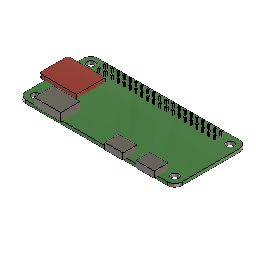
PiZero (Autodesk Fusion 360 design; units mm, degrees)
Autodesk Fusion 360 part; units mm, degrees
sketch "Skizze1" plane through (0, 0, 0) normal (0, 0, 1) x (1, 0, 0)
  line L0 (0, 0) -> (65, 0)
  line L1 (65, 0) -> (65, 30)
  line L2 (65, 30) -> (0, 30)
  line L3 (0, 30) -> (0, 0)
  dimension "d1" = 65
  dimension "d2" = 30
  constraint horizontal L0
  constraint vertical L1
  constraint horizontal L2
  constraint vertical L3
  constraint coincident L0.start L3.end
  measures "d1" distance of L0.start L0.end
  measures "d2" distance of L0.end L1.end
extrude "Extrusion1" add sketch "Skizze1" along normal blind 1.3
fillet "Abrundung1" radius 3 4 edges at (65, 0, 0.65) (0, 0, 0.65) (0, 30, 0.65) (65, 30, 0.65)
sketch "Skizze2" plane through (0, 0, 1.3) normal (0, 0, 1) x (-1, 0, 0)
  arc A0 (-65, -27) -> (-62, -30) centre (-62, -27) ccw
  line L0 (-62, -30) -> (-3, -30)
  arc A1 (-3, -30) -> (0, -27) centre (-3, -27) ccw
  line L1 (0, -27) -> (0, -3)
  arc A2 (0, -3) -> (-3, 0) centre (-3, -3) ccw
  line L2 (-3, 0) -> (-62, 0)
  arc A3 (-62, 0) -> (-65, -3) centre (-62, -3) ccw
  line L3 (-65, -3) -> (-65, -27)
  line L4 (2.5, -23) -> (-13, -23)
  line L5 (-13, -23) -> (-13, -11)
  line L6 (-13, -11) -> (2.5, -11)
  line L7 (2.5, -11) -> (2.5, -23)
  dimension "d7" = 12
  dimension "d8" = 15.5
  dimension "d9" = 7
  dimension "d10" = 2.5
  constraint horizontal L4
  constraint vertical L5
  constraint horizontal L6
  constraint vertical L7
  measures "d7" distance of L4.end L5.end
  measures "d8" distance of L5.end L6.end
  measures "d9" distance of L0 L4
  measures "d10" distance of L1 L7
extrude "Extrusion2" add sketch "Skizze2" along normal blind 1.5 contours L1 L4 L5 L6 | L1 L4 L6 L7
fillet "Abrundung2" radius 1 2 edges at (-2.5, 11, 2.05) (-2.5, 23, 2.05)
sketch "Skizze3" plane through (0, 0, 1.3) normal (0, 0, 1) x (-1, 0, 0)
  line L0 (-13, -11) -> (0, -11)
  line L1 (0, -11) -> (0, -3)
  arc A0 (0, -3) -> (-3, 0) centre (-3, -3) ccw
  line L2 (-3, 0) -> (-62, 0)
  arc A1 (-62, 0) -> (-65, -3) centre (-62, -3) ccw
  line L3 (-65, -3) -> (-65, -27)
  arc A2 (-65, -27) -> (-62, -30) centre (-62, -27) ccw
  line L4 (-62, -30) -> (-3, -30)
  arc A3 (-3, -30) -> (0, -27) centre (-3, -27) ccw
  line L5 (0, -27) -> (0, -23)
  line L6 (0, -23) -> (-13, -23)
  line L7 (-13, -23) -> (-13, -11)
  line L8 (-7, -7.5) -> (-18, -7.5)
  line L9 (-18, -7.5) -> (-18, 0.5)
  line L10 (-18, 0.5) -> (-7, 0.5)
  line L11 (-7, 0.5) -> (-7, -7.5)
  dimension "d15" = 8
  dimension "d16" = 11
  dimension "d17" = 7
  dimension "d18" = 0.5
  constraint horizontal L8
  constraint vertical L9
  constraint horizontal L10
  constraint vertical L11
  measures "d15" distance of L8.end L9.end
  measures "d16" distance of L9.end L10.end
  measures "d17" distance of L1 L11
  measures "d18" distance of L2 L10
extrude "Extrusion3" add sketch "Skizze3" along normal blind 3.2 contours L2 L8 L9 L11 | L2 L9 L10 L11
sketch "Skizze4" plane through (0, 0, 1.3) normal (0, 0, 1) x (-1, 0, 0)
  line L0 (-18, -7.5) -> (-18, 0)
  line L1 (-18, 0) -> (-62, 0)
  arc A0 (-62, 0) -> (-65, -3) centre (-62, -3) ccw
  line L2 (-65, -3) -> (-65, -27)
  arc A1 (-65, -27) -> (-62, -30) centre (-62, -27) ccw
  line L3 (-62, -30) -> (-3, -30)
  arc A2 (-3, -30) -> (0, -27) centre (-3, -27) ccw
  line L4 (0, -27) -> (0, -23)
  line L5 (0, -23) -> (-13, -23)
  line L6 (-13, -23) -> (-13, -11)
  line L7 (-13, -11) -> (0, -11)
  line L8 (0, -11) -> (0, -3)
  arc A3 (0, -3) -> (-3, 0) centre (-3, -3) ccw
  line L9 (-3, 0) -> (-7, 0)
  line L10 (-7, 0) -> (-7, -7.5)
  line L11 (-7, -7.5) -> (-18, -7.5)
  line L12 (-37.4, -4.2) -> (-44.9, -4.2)
  line L13 (-44.9, -4.2) -> (-44.9, 1.5)
  line L14 (-44.9, 1.5) -> (-37.4, 1.5)
  line L15 (-37.4, 1.5) -> (-37.4, -4.2)
  dimension "d21" = 7.5
  dimension "d22" = 5.7
  dimension "d23" = 37.4
  dimension "d24" = 1.5
  constraint horizontal L12
  constraint vertical L13
  constraint horizontal L14
  constraint vertical L15
  measures "d21" distance of L13.end L14.end
  measures "d22" distance of L12.end L13.end
  measures "d23" distance of L8 L15
  measures "d24" distance of L1 L14
extrude "Extrusion4" add sketch "Skizze4" along normal blind 2.6 contours L1 L12 L13 L15 | L1 L13 L14 L15
pattern_linear "R-Anordnung1" count 2 spacing 13 along (1, 0, 0) of "Extrusion4"
sketch "Skizze5" plane through (0, 0, 1.3) normal (0, 0, 1) x (-1, 0, 0)
  line L0 (-50.4, 0) -> (-50.4, -4.2)
  line L1 (-50.4, -4.2) -> (-57.9, -4.2)
  line L2 (-57.9, -4.2) -> (-57.9, 0)
  line L3 (-57.9, 0) -> (-62, 0)
  arc A0 (-62, 0) -> (-65, -3) centre (-62, -3) ccw
  line L4 (-65, -3) -> (-65, -27)
  arc A1 (-65, -27) -> (-62, -30) centre (-62, -27) ccw
  line L5 (-62, -30) -> (-3, -30)
  arc A2 (-3, -30) -> (0, -27) centre (-3, -27) ccw
  line L6 (0, -27) -> (0, -23)
  line L7 (0, -23) -> (-13, -23)
  line L8 (-13, -23) -> (-13, -11)
  line L9 (-13, -11) -> (0, -11)
  line L10 (0, -11) -> (0, -3)
  arc A3 (0, -3) -> (-3, 0) centre (-3, -3) ccw
  line L11 (-3, 0) -> (-7, 0)
  line L12 (-7, 0) -> (-7, -7.5)
  line L13 (-7, -7.5) -> (-18, -7.5)
  line L14 (-18, -7.5) -> (-18, 0)
  line L15 (-18, 0) -> (-37.4, 0)
  line L16 (-37.4, 0) -> (-37.4, -4.2)
  line L17 (-37.4, -4.2) -> (-44.9, -4.2)
  line L18 (-44.9, -4.2) -> (-44.9, 0)
  line L19 (-44.9, 0) -> (-50.4, 0)
  point P0 (-3.5, -26.5)
  point P1 (-61.5, -26.5)
  point P2 (-61.5, -3.5)
  point P3 (-3.5, -3.5)
  dimension "d31" = 58
  dimension "d32" = 58
  dimension "d33" = 3.5
  dimension "d34" = 3.5
  dimension "d35" = 3.5
  dimension "d36" = 3.5
  dimension "d37" = 3.5
  dimension "d38" = 3.5
  measures "d31" distance of P2 P3
  measures "d32" distance of P0 P1
  measures "d33" distance of L4 P2
  measures "d34" distance of L4 P1
  measures "d35" distance of L5 P1
  measures "d36" distance of L5 P0
  measures "d37" distance of L11 P3
  measures "d38" distance of L3 P2
hole "Bohrung1" at (3.5, 26.5, 1.3) at (61.5, 26.5, 1.3) at (61.5, 3.5, 1.3) at (3.5, 3.5, 1.3) direction (0, 0, -1) diameter 3.2 end through all
sketch "Skizze7" plane through (0, 0, 0) normal (0, 0, -1) x (1, 0, 0)
  circle A0 centre (61.5, -3.5) radius 1.6
  circle A1 centre (3.5, -26.5) radius 1.6
  circle A2 centre (61.5, -26.5) radius 1.6
  circle A3 centre (3.5, -3.5) radius 1.6
  arc A4 (62, -30) -> (65, -27) centre (62, -27) ccw
  line L0 (65, -27) -> (65, -3)
  arc A5 (65, -3) -> (62, 0) centre (62, -3) ccw
  line L1 (62, 0) -> (3, 0)
  arc A6 (3, 0) -> (0, -3) centre (3, -3) ccw
  line L2 (0, -3) -> (0, -27)
  arc A7 (0, -27) -> (3, -30) centre (3, -27) ccw
  line L3 (3, -30) -> (62, -30)
  line L4 (7.1, -23.96) -> (57.9, -23.96)
  line L5 (57.9, -23.96) -> (57.9, -29.04)
  line L6 (57.9, -29.04) -> (7.1, -29.04)
  line L7 (7.1, -29.04) -> (7.1, -23.96)
  dimension "d42" = 50.8
  dimension "d43" = 5.08
  dimension "d44" = 3.6
  dimension "d45" = 3.6
  dimension "d46" = 0.96
  constraint horizontal L4
  constraint vertical L5
  constraint horizontal L6
  constraint vertical L7
  measures "d42" distance of L5.end L6.end
  measures "d43" distance of L4.end L5.end
  measures "d44" distance of A2.centre L5
  measures "d45" distance of A1.centre L7
  measures "d46" distance of L3 L6
extrude "Extrusion5" add sketch "Skizze7" along normal blind 2.5 contours L4 L5 L6 L7
fillet "Abrundung3" radius 1 4 edges at (7.1, 29.04, -1.25) (7.1, 23.96, -1.25) (57.9, 23.96, -1.25) (57.9, 29.04, -1.25)
sketch "Skizze8" plane through (0, 0, -2.5) normal (0, 0, -1) x (1, 0, 0)
  arc A0 (56.9, -29.04) -> (57.9, -28.04) centre (56.9, -28.04) ccw
  line L0 (57.9, -28.04) -> (57.9, -24.96)
  arc A1 (57.9, -24.96) -> (56.9, -23.96) centre (56.9, -24.96) ccw
  line L1 (56.9, -23.96) -> (8.1, -23.96)
  arc A2 (8.1, -23.96) -> (7.1, -24.96) centre (8.1, -24.96) ccw
  line L2 (7.1, -24.96) -> (7.1, -28.04)
  arc A3 (7.1, -28.04) -> (8.1, -29.04) centre (8.1, -28.04) ccw
  line L3 (8.1, -29.04) -> (56.9, -29.04)
  line L4 (7.97, -24.83) -> (8.77, -24.83)
  line L5 (8.77, -24.83) -> (8.77, -25.63)
  line L6 (8.77, -25.63) -> (7.97, -25.63)
  line L7 (7.97, -25.63) -> (7.97, -24.83)
  line L8 (0, -27) -> (0, -3)
  dimension "d51" = 0.8
  dimension "d52" = 0.8
  dimension "d54" = 0.87
  dimension "d55" = 0.87
  constraint horizontal L4
  constraint vertical L5
  constraint horizontal L6
  constraint vertical L7
  measures "d51" distance of L5.end L6.end
  measures "d52" distance of L4.start L6.end
  measures "d54" distance of L2 L6.end
  measures "d55" distance of L1 L4
extrude "Extrusion6" add sketch "Skizze8" along normal mid plane 11.2 contours L4 L5 L6 L7
chamfer "Fase1" distance 0.15 angle 45 16 edges at (7.97, 25.63, -5.3) (7.97, 24.83, -5.3) (8.77, 24.83, -5.3) (8.77, 25.63, -5.3) (8.77, 25.23, -8.1) (8.37, 24.83, -8.1) (7.97, 25.23, -8.1) (8.37, 25.63, -8.1) (7.97, 25.63, 2.2) (7.97, 24.83, 2.2) (8.77, 24.83, 2.2) (8.77, 25.63, 2.2) (8.37, 25.63, 3.1) (8.37, 24.83, 3.1) (8.77, 25.23, 3.1) (7.97, 25.23, 3.1)
pattern_linear "R-Anordnung2" count 20 spacing 2.54 along (1, 0, 0) count 2 spacing 2.54 along (0, 1, 0) of "Extrusion6", "Fase1"
equation "d42 = ( 20 * 2.54 ) * 1 mm"
equation "d44 = 29 mm - d42 / 2"
equation "d46 = 3.5 mm - 2.54 mm"
equation "d54 = 1.27 mm - 0.4 mm"
equation "d55 = 1.27 mm - 0.4 mm"
